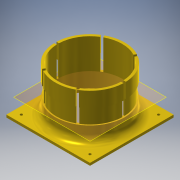
# Autodesk Inventor part: Cup_Dispenser_Fixture
Saved by Autodesk Inventor 2016 (Build 200138000, 138)
## iProperties
Created: 2015-07-09
Part Number: Cup_Dispenser_Fixture
Material: Generic
Document SubType Name: Modeling
Designer: marku
Density: 1 g/cm^3
Appearance: Glossy - Gold
Author: marku
Autodesk Inventor part; units mm, degrees
ref_plane "YZ Plane" through (0, 0, 0) normal (1, 0, 0) x (0, 1, 0)
ref_plane "XZ Plane" through (0, 0, 0) normal (0, 1, 0) x (-1, 0, 0)
ref_plane "XY Plane" through (0, 0, 0) normal (0, 0, 1) x (1, 0, 0)
sketch "Sketch1" plane through (0, 0, 0) normal (0, 0, 1) x (1, 0, 0)
  circle A0 centre (-41, -93.7922) radius 1.5 projected
  circle A1 centre (41, -93.7922) radius 1.5 projected
  circle A2 centre (-41, 88.2078) radius 1.5 projected
  circle A3 centre (41, 6.2078) radius 1.5 projected
  circle A4 centre (41, 88.2078) radius 1.5 projected
  circle A5 centre (-41, 6.2078) radius 1.5 projected
  circle A6 centre (41, -11.7922) radius 1.5 projected
  circle A7 centre (-41, -11.7922) radius 1.5 projected
  circle A8 centre (0, -52.7922) radius 47 projected
  circle A9 centre (0, 47.2078) radius 47 projected
  line L0 (-50, 97.2078) -> (-50, -92.7922) projected
  arc A10 (-50, -92.7922) -> (-40, -102.7922) centre (-40, -92.7922) ccw projected
  line L1 (-40, -102.7922) -> (40, -102.7922) projected
  arc A11 (40, -102.7922) -> (50, -92.7922) centre (40, -92.7922) ccw projected
  line L2 (50, -92.7922) -> (50, 97.2078) projected
  line L3 (50, 97.2078) -> (-50, 97.2078) projected
  line L4 (-50, -2.7922) -> (50, -2.7922)
  line L5 (50, -2.7922) -> (50, 97.2078)
  line L6 (50, 97.2078) -> (-50, 97.2078)
  line L7 (-50, 97.2078) -> (-50, -2.7922)
  line L8 (-50, -2.7922) -> (50, 97.2078) construction
  line L9 (50, -2.7922) -> (-50, 97.2078) construction
  circle A12 centre (0, 47.2078) radius 37.5
  point P0 (0, 0)
  dimension "d3" = 75
  constraints: 12 end point, 3 midpoint, 2 parallel, 1 centre point, 1 coincident, 1 horizontal, 1 perpendicular
  measures "d3" diameter of A12
extrude "Extrusion1" add sketch "Sketch1" along normal blind 3 contours A9 | L3 L2 L4 L0
sketch "Sketch3" plane through (0, 0, 3) normal (0, 0, 1) x (1, 0, 0)
  circle A0 centre (0, 47.2078) radius 37.5 construction
  circle A1 centre (0, 47.2078) radius 38.5
  circle A2 centre (0, 47.2078) radius 41.5
  point P0 (0, 0)
  dimension "d4" = 77
  dimension "d5" = 3
  constraints: 2 centre point, 1 coincident
  measures "d4" diameter of A1
  measures "d5" radial gap between concentric circles of A1 A2
extrude "Extrusion2" add sketch "Sketch3" along normal blind 54
ref_plane "Work Plane1" through (0, 47.2078, 21) normal (0, 0, 1) x (1, 0, 0)
sketch "Sketch4" plane through (0, 47.2078, 21) normal (0, 0, 1) x (1, 0, 0)
  circle A0 centre (0, 0) radius 38.5 construction
  circle A1 centre (0, 0) radius 41.5 projected
  circle A2 centre (0, 0) radius 40
  point P0 (0, -47.2078)
  dimension "d9" = 1.5
  constraints: 1 centre point
  measures "d9" radial gap between concentric circles of A1 A2
extrude "Extrusion3" cut sketch "Sketch4" along normal blind 18
sketch "Sketch5" plane through (0, 47.2078, 57) normal (0, 0, 1) x (1, 0, 0)
  circle A0 centre (0, 0) radius 38.5 projected
  circle A1 centre (0, 0) radius 41.5 projected
  line L0 (0, 0) -> (-53, 0) construction
  line L1 (0, 0) -> (-41.4747, -1.4483)
  circle A2 centre (0, 0) radius 41.5 projected
  line L2 (0, 0) -> (-41.4747, 1.4483)
  point P0 (0, -47.2078)
  dimension "d12" = 4
  constraints: 6 end point, 4 point on circle, 1 horizontal, 1 other
  measures "d12" angle of L2 L1
extrude "Extrusion4" cut sketch "Sketch5" against normal up to surface (36 mm away) contours L2 L1 A0 | A0 L1 A1 L2 picked at (-25.658, -0.5972) picked at (-40.4973, 0.1493)
pattern_circular "Circular Pattern1" count 6 over 360 about axis through (0, 47.2078, 3) along (0, 0, 1) of "Extrusion4"
fillet "Fillet1" radius 9 1 edges at (-41.5, 47.2078, 3)
equation "\"d0\" = thickness"
equation "\"d5\" = thickness"
equation "\"d6\" = fixture_height"
equation "\"d9\" = 0.5 * thickness"
equation "\"d10\" = 0.333333 * fixture_height"
equation "\"d18\" = 3 * thickness"
equation "\"thickness\" = 3"
equation "\"fixture_height\" = 18 * thickness"
equation "\"d8\" = -0.666667 * fixture_height"
body "Solid1"
